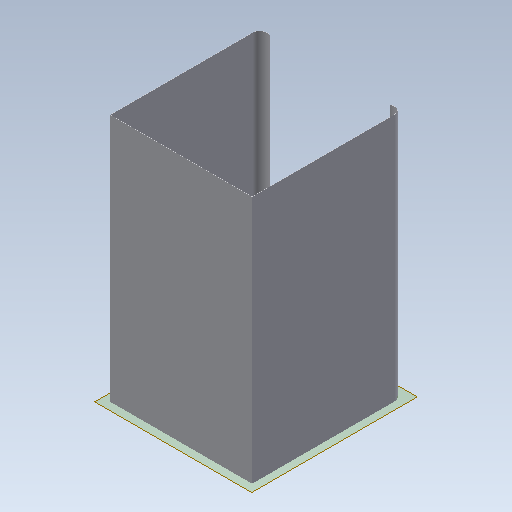
# Autodesk Inventor part: Standard
Saved by Autodesk Inventor 2020.3 (Build 243373000, 373)
## iProperties
RuleStatus: InUse
AfterDocSave0: file://Part Number Cleaner
Created: 2023-03-03
Material: PET, WHITE
Catalog Web Link: https://www.janelia.org/
Vendor: HHMI: JRC - jET
Document SubType Name: Modeling
Designer: jalala
Density: 1.41 g/cm^3
Appearance: Plastic (White)
DESIGN DEPARTMENT: HHMI: JRC - jET
ALTERED ITEM PART NUMBER: N/A
ALTERED ITEM VENDOR: N/A
ALTERED ITEM DESCRIPTION: N/A
Title: Standard
Author: jalala
Revision Number: 0
Autodesk Inventor part; units mm, degrees
ref_plane "YZ Plane" through (0, 0, 0) normal (1, 0, 0) x (0, 1, 0)
ref_plane "XZ Plane" through (0, 0, 0) normal (0, 1, 0) x (-1, 0, 0)
ref_plane "Work Plane1" through (0, 0, -1.5875) normal (0, -1, 0) x (1, 0, 0)
sketch "Sketch1" plane through (0, 0, -1.5875) normal (0, -1, 0) x (1, 0, 0)
  line L0 (28.956, 30.5435) -> (28.956, -27.6225) projected
  line L1 (-28.956, 30.5435) -> (28.956, 30.5435) projected
  line L2 (-28.956, -27.6225) -> (-28.956, 30.5435) projected
  circle A0 centre (26.035, -27.6225) radius 1.4732 construction
  circle A1 centre (-26.035, -27.6225) radius 1.4732 construction
  arc A2 (24.5745, -30.1522) -> (28.956, -27.6225) centre (26.035, -27.6225) ccw
  arc A3 (-28.956, -27.6225) -> (-24.5745, -30.1522) centre (-26.035, -27.6225) ccw
  line L3 (29.083, -27.6225) -> (29.083, 30.6705)
  line L4 (29.083, 30.6705) -> (-29.083, 30.6705)
  line L5 (-29.083, 30.6705) -> (-29.083, -27.6225)
  arc A4 (24.511, -30.2621) -> (29.083, -27.6225) centre (26.035, -27.6225) ccw
  arc A5 (-29.083, -27.6225) -> (-24.511, -30.2621) centre (-26.035, -27.6225) ccw
  line L6 (-26.035, -27.6225) -> (-24.511, -30.2621) construction
  line L7 (-24.5745, -30.1522) -> (-24.511, -30.2621)
  line L8 (-26.035, -27.6225) -> (-26.035, -29.4353) construction
  line L9 (26.035, -27.6225) -> (24.511, -30.2621) construction
  line L10 (26.035, -27.6225) -> (26.035, -29.6779) construction
  line L11 (24.511, -30.2621) -> (24.5745, -30.1522)
  point P0 (0, 1.5875)
  dimension "d0" = 0.127
  dimension "d1" = 0.127
  dimension "d3" = 0.127
  dimension "d4" = 0.127
  dimension "d5" = 0.127
  dimension "d8" = 30
  dimension "d9" = 30
  constraints: 18 end point, 8 point on circle, 4 centre point, 4 coincident, 3 vertical, 2 parallel, 2 point on line, 1 collinear
  measures "d0" distance between parallel lines of L0 L3
  measures "d1" distance between parallel lines of L1 L4
  measures "d3" distance between parallel lines of L2 L5
  measures "d4" radial gap between concentric circles of A3 A5
  measures "d5" radial gap between concentric circles of A2 A4
  measures "d8" angle of L6 L8
  measures "d9" angle of L9 L10
ref_plane "Work Plane2" through (-29.21, 101.6, -32.385) normal (0, 1, 0) x (0, 0, 1)
extrude "Extrusion1" add sketch "Sketch1" against normal blind 101.6
body "Solid1"
